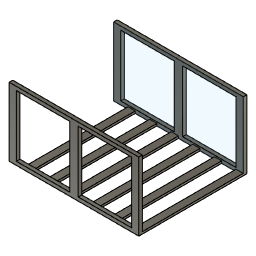
Suporte (Autodesk Fusion 360 design; units mm, degrees)
Autodesk Fusion 360 part; units mm, degrees
sketch "Esboço1" plane through (0, 0, 0) normal (0, 0, 1) x (1, 0, 0)
  line L0 (90, -75) -> (-90, -75)
  line L1 (-90, -75) -> (-90, 75)
  line L2 (-90, 75) -> (90, 75)
  line L3 (90, 75) -> (90, -75)
  line L4 (90, -75) -> (-90, 75) construction
  line L5 (-90, -75) -> (90, 75) construction
  dimension "d1" = 180
  dimension "d2" = 150
  constraint horizontal L0
  constraint perpendicular L0 L1
  constraint parallel L0 L2
  constraint parallel L1 L3
  constraint coincident L4 origin
  constraint coincident L5 origin
  measures "d1" distance of L1.end L2.end
  measures "d2" distance of L0.end L1.end
extrude "Extrusão1" add sketch "Esboço1" along normal blind 95
sketch "Esboço2" plane through (0, 0, 95) normal (0, 0, 1) x (-1, 0, 0)
  line L0 (-90, -75) -> (90, -75)
  line L1 (90, -75) -> (90, 75)
  line L2 (90, 75) -> (-90, 75)
  line L3 (-90, 75) -> (-90, -75)
  line L4 (-95, 70) -> (95, 70)
  line L5 (95, 70) -> (95, -70)
  line L6 (95, -70) -> (-95, -70)
  line L7 (-95, -70) -> (-95, 70)
  line L8 (-95, 70) -> (95, -70) construction
  line L9 (95, 70) -> (-95, -70) construction
  dimension "d5" = 190
  dimension "d6" = 140
  constraint horizontal L4
  constraint perpendicular L4 L5
  constraint parallel L4 L6
  constraint parallel L5 L7
  constraint coincident L8 origin
  constraint coincident L9 origin
  measures "d5" distance of L5.end L6.end
  measures "d6" distance of L4.end L5.end
extrude "Extrusão2" cut sketch "Esboço2" against normal blind 92 contours L1 L3 L4 L6
sketch "Esboço3" plane through (0, 0, 3) normal (0, 0, 1) x (-1, 0, 0)
  line L0 (-90, 70) -> (-90, -70)
  line L1 (-90, -70) -> (90, -70)
  line L2 (90, -70) -> (90, 70)
  line L3 (90, 70) -> (-90, 70)
  line L4 (-80, 70) -> (-60, 70)
  line L5 (-60, 70) -> (-60, -70)
  line L6 (-60, -70) -> (-80, -70)
  line L7 (-80, -70) -> (-80, 70)
  line L8 (-50, 70) -> (-30, 70)
  line L9 (-30, 70) -> (-30, -70)
  line L10 (-30, -70) -> (-50, -70)
  line L11 (-50, -70) -> (-50, 70)
  line L12 (-20, 70) -> (0, 70)
  line L13 (0, 70) -> (0, -70)
  line L14 (0, -70) -> (-20, -70)
  line L15 (-20, -70) -> (-20, 70)
  line L16 (10, 70) -> (30, 70)
  line L17 (30, 70) -> (30, -70)
  line L18 (30, -70) -> (10, -70)
  line L19 (10, -70) -> (10, 70)
  line L20 (40, 70) -> (60, 70)
  line L21 (60, 70) -> (60, -70)
  line L22 (60, -70) -> (40, -70)
  line L23 (40, -70) -> (40, 70)
  line L24 (70, 70) -> (80, 70)
  line L25 (80, 70) -> (80, -70)
  line L26 (80, -70) -> (70, -70)
  line L27 (70, -70) -> (70, 70)
  constraint horizontal L4
  constraint vertical L5
  constraint horizontal L6
  constraint vertical L7
  constraint coincident L1 L5.end
  constraint coincident L3 L4.start
  constraint horizontal L8
  constraint vertical L9
  constraint horizontal L10
  constraint vertical L11
  constraint coincident L1 L9.end
  constraint coincident L3 L8.start
  constraint horizontal L12
  constraint vertical L13
  constraint horizontal L14
  constraint vertical L15
  constraint midpoint L1 L13.end
  constraint coincident L3 L12.start
  constraint horizontal L16
  constraint vertical L17
  constraint horizontal L18
  constraint vertical L19
  constraint coincident L1 L17.end
  constraint coincident L3 L16.start
  constraint horizontal L20
  constraint vertical L21
  constraint horizontal L22
  constraint vertical L23
  constraint coincident L1 L21.end
  constraint coincident L3 L20.start
  constraint horizontal L24
  constraint vertical L25
  constraint horizontal L26
  constraint vertical L27
  constraint coincident L1 L25.end
  constraint coincident L3 L24.start
extrude "Extrusão3" cut sketch "Esboço3" against normal blind 10 contours L1 L3 L4 L5 L6 L7 | L1 L3 L8 L9 L10 L11 | L1 L3 L12 L13 L14 L15 | L1 L3 L16 L17 L18 L19 | L1 L3 L20 L21 L22 L23 | L1 L3 L24 L25 L26 L27
delete_face "Excluir face1" 1 faces at (-83.3333, 23.3333, 3)
sketch "Esboço4" plane through (0, 0, 0) normal (0, 1, 0) x (1, 0, 0)
sketch "Esboço5" plane through (0, 0, 0) normal (0, 1, 0) x (1, 0, 0)
move_body "Mover1" bodies 1 to x (1, 0, 0) y (0, 1, 0) z (0, 0, 1) at (0, 0, -40)
sketch "Esboço6" plane through (0, 70, 0) normal (0, -1, 0) x (1, 0, 0)
  line L0 (90, 55) -> (-90, 55)
  line L1 (-90, 55) -> (-90, -40)
  line L2 (-90, -40) -> (-70, -40)
  line L3 (-70, -40) -> (-70, -37)
  line L4 (-70, -37) -> (-60, -37)
  line L5 (-60, -37) -> (-60, -40)
  line L6 (-60, -40) -> (-40, -40)
  line L7 (-40, -40) -> (-40, -37)
  line L8 (-40, -37) -> (-30, -37)
  line L9 (-30, -37) -> (-30, -40)
  line L10 (-30, -40) -> (-10, -40)
  line L11 (-10, -40) -> (-10, -37)
  line L12 (-10, -37) -> (0, -37)
  line L13 (0, -37) -> (0, -40)
  line L14 (0, -40) -> (20, -40)
  line L15 (20, -40) -> (20, -37)
  line L16 (20, -37) -> (30, -37)
  line L17 (30, -37) -> (30, -40)
  line L18 (30, -40) -> (50, -40)
  line L19 (50, -40) -> (50, -37)
  line L20 (50, -37) -> (60, -37)
  line L21 (60, -37) -> (60, -40)
  line L22 (60, -40) -> (80, -40)
  line L23 (80, -40) -> (80, -37)
  line L24 (80, -37) -> (90, -37)
  line L25 (90, -37) -> (90, 55)
sketch "Esboço7" plane through (0, -75, 0) normal (0, -1, 0) x (1, 0, 0)
  line L0 (-90, -40) -> (90, -40)
  line L1 (90, -40) -> (90, 55)
  line L2 (90, 55) -> (-90, 55)
  line L3 (-90, 55) -> (-90, -40)
  line L4 (-80, 50) -> (-5.8421, 50)
  line L5 (-5.8421, 50) -> (-5.8421, -35.0525)
  line L6 (-5.8421, -35.0525) -> (-80, -35.0525)
  line L7 (-80, -35.0525) -> (-80, 50)
  constraint horizontal L4
  constraint vertical L5
  constraint horizontal L6
  constraint vertical L7
extrude "Extrusão4" cut sketch "Esboço7" against normal blind 200 contours L4 L5 L6 L7
sketch "Esboço8" plane through (0, -75, 0) normal (0, -1, 0) x (1, 0, 0)
  line L0 (-5.8421, 50) -> (-5.8421, -35.0525)
  line L1 (-5.8421, -35.0525) -> (-80, -35.0525)
  line L2 (-80, -35.0525) -> (-80, 50)
  line L3 (-80, 50) -> (-5.8421, 50)
  line L4 (-90, -40) -> (90, -40)
  line L5 (90, -40) -> (90, 55)
  line L6 (90, 55) -> (-90, 55)
  line L7 (-90, 55) -> (-90, -40)
  line L8 (5.8421, 50) -> (80.0001, 50)
  line L9 (80.0001, 50) -> (80.0001, -35.053)
  line L10 (80.0001, -35.053) -> (5.8421, -35.053)
  line L11 (5.8421, -35.053) -> (5.8421, 50)
  dimension "d17" = 74.158
  dimension "d18" = 85.053
  constraint horizontal L8
  constraint vertical L9
  constraint horizontal L10
  constraint vertical L11
  measures "d17" distance of L8.start L8.end
  measures "d18" distance of L8.end L9.end
extrude "Extrusão5" cut sketch "Esboço8" against normal blind 190 contours L8 L9 L10 L11
